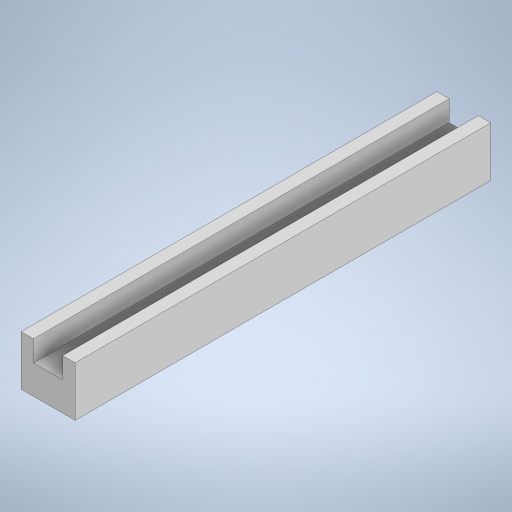
# Autodesk Inventor part: Part6-01
Saved by Autodesk Inventor 2023.2 (Build 272271000, 271)
## iProperties
Created: 2022-12-21
Part Number: Part6-01
Material: Generic
Document SubType Name: Modeling
Designer: Felipe Coquito
Density: 1 g/cm^3
Appearance: Default
Author: Felipe Coquito
Autodesk Inventor part; units mm, degrees
ref_plane "YZ Plane" through (0, 0, 0) normal (1, 0, 0) x (0, 1, 0)
ref_plane "XZ Plane" through (0, 0, 0) normal (0, 1, 0) x (-1, 0, 0)
ref_plane "XY Plane" through (0, 0, 0) normal (0, 0, 1) x (1, 0, 0)
sketch "Sketch1" plane through (0, 0, 0) normal (0, 0, 1) x (1, 0, 0)
  line L0 (0, 0) -> (-13, 0)
  line L1 (-13, 0) -> (-13, 12)
  line L2 (-13, 12) -> (-10, 12)
  line L3 (-10, 12) -> (-10, 7)
  line L4 (-10, 7) -> (-3, 7)
  line L5 (-3, 7) -> (-3, 12)
  line L6 (-3, 12) -> (0, 12)
  line L7 (0, 12) -> (0, 0)
  dimension "d0" = 13
  dimension "d1" = 3
  dimension "d2" = 3
  dimension "d3" = 12
  dimension "d4" = 5
  constraints: 16 end point, 6 perpendicular, 2 point on line, 1 horizontal
  measures "d0" distance of L0.start L0.end
  measures "d1" distance of L1.end L2.end
  measures "d2" distance of L5.end L6.end
  measures "d3" distance of L6.end L0.start
  measures "d4" distance of L3.end L2.end
extrude "Extrusion1" add sketch "Sketch1" along normal blind 100
body "Solid1"
